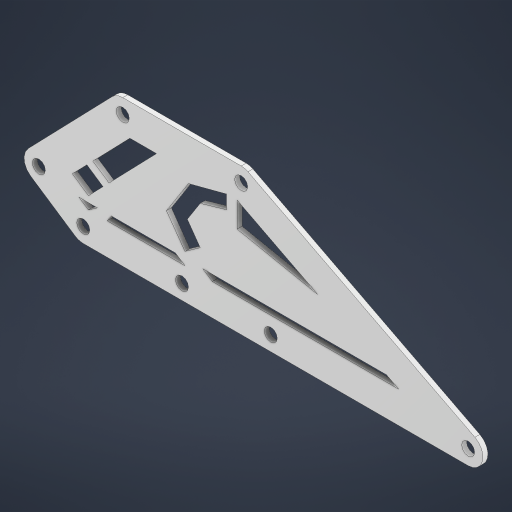
# Autodesk Inventor part: battery_mount_plate
Saved by Autodesk Inventor 2024 (Build 280153000, 153)
## iProperties
Created: 2023-11-22
Part Number: battery_mount_plate
Material: Acetal Resin, White
Document SubType Name: Modeling
Designer: avere
Density: 1.425 g/cm^3
Appearance: Smooth - White
Author: avere
Autodesk Inventor part; units mm, degrees
ref_plane "YZ Plane" through (0, 0, 0) normal (1, 0, 0) x (0, 1, 0)
ref_plane "XZ Plane" through (0, 0, 0) normal (0, 1, 0) x (-1, 0, 0)
ref_plane "XY Plane" through (0, 0, 0) normal (0, 0, 1) x (1, 0, 0)
sketch "Sketch1" plane through (0, 0, 0) normal (0, 0, 1) x (1, 0, 0)
  circle A0 centre (-66.446, -8.2221) radius 2.0955
  arc A1 (-69.8715, -4.9134) -> (-69.0877, -12.1847) centre (-66.446, -8.2221) ccw
  circle A2 centre (-39.4585, 19.7179) radius 2.0955
  circle A3 centre (-1.3585, 19.7179) radius 2.0955
  arc A4 (-39.4585, 24.4804) -> (-42.884, 23.0266) centre (-39.4585, 19.7179) ccw
  arc A5 (0.8155, 23.9553) -> (-1.3585, 24.4804) centre (-1.3585, 19.7179) ccw
  line L0 (-39.4585, 24.4804) -> (-1.3585, 24.4804)
  line L1 (-69.8715, -4.9134) -> (-42.884, 23.0266)
  circle A6 centre (-52.1585, -17.7471) radius 2.0955
  arc A7 (-54.8002, -21.7097) -> (-52.1585, -22.5096) centre (-52.1585, -17.7471) ccw
  circle A8 centre (-20.4085, -17.7471) radius 2.0955
  circle A9 centre (8.1665, -17.7471) radius 2.0955
  circle A10 centre (71.6665, -17.7471) radius 2.0955
  arc A11 (71.6665, -22.5096) -> (73.8405, -13.5097) centre (71.6665, -17.7471) ccw
  line L2 (0.8155, 23.9553) -> (73.8405, -13.5097)
  line L3 (-52.1585, -22.5096) -> (71.6665, -22.5096)
  line L4 (-54.8002, -21.7097) -> (-69.0877, -12.1847)
  line L5 (-28.575, 14.3204) -> (-37.1677, 14.3204)
  line L6 (-53.5722, -10.3176) -> (-50.5242, -12.3496)
  line L7 (-19.456, -12.3496) -> (-22.504, -10.3176)
  line L8 (-10.6535, -12.3496) -> (-13.7015, -10.3176)
  line L9 (-13.7015, -10.3176) -> (45.361, -10.3176)
  line L10 (-13.7015, -10.3176) -> (45.361, -10.3176) construction
  line L11 (-44.45, -12.3496) -> (-19.456, -12.3496)
  line L12 (-10.6535, -12.3496) -> (49.3216, -12.3496)
  line L13 (-50.5242, -12.3496) -> (-47.6187, -10.3176)
  line L14 (-44.45, -12.3496) -> (-43.0953, -10.3176)
  line L15 (-53.5722, -10.3176) -> (-47.6187, -10.3176)
  line L16 (-43.0953, -10.3176) -> (-22.504, -10.3176)
  line L17 (-53.5722, -10.3176) -> (-47.6187, -10.3176) construction
  line L18 (-43.0953, -10.3176) -> (-22.504, -10.3176) construction
  line L19 (-55.6904, -4.856) -> (-50.4835, -8.3613)
  line L20 (-51, 0) -> (-45.7931, -3.5053)
  line L21 (-49.0715, 1.9965) -> (-43.8646, -1.5088)
  line L22 (-50.4835, -8.3613) -> (-45.7931, -3.5053)
  line L23 (-43.8646, -1.5088) -> (-28.575, 14.3204)
  line L24 (-37.1677, 14.3204) -> (-49.0715, 1.9965)
  line L25 (-51, 0) -> (-55.6904, -4.856)
  line L26 (-2.6623, 14.3204) -> (-2.6623, 6.2412)
  line L27 (-2.6623, 6.2412) -> (23.3297, 0.9854)
  line L28 (23.3297, 0.9854) -> (-2.6623, 14.3204)
  line L29 (49.3216, -12.3496) -> (45.361, -10.3176)
  line L30 (-6.0786, 14.3204) -> (-18.313, 11.1125)
  line L31 (-18.313, 11.1125) -> (-25.4, 0)
  line L32 (-25.4, 0) -> (-19.456, -8.3613)
  line L33 (-19.456, -8.3613) -> (-14.5251, -4.856)
  line L34 (-14.5251, -4.856) -> (-18.6777, 0.9854)
  line L35 (-18.6777, 0.9854) -> (-14.5251, 7.4968)
  line L36 (-14.5251, 7.4968) -> (-6.0786, 9.9421)
  line L37 (-6.0786, 9.9421) -> (-6.0786, 14.3204)
  point P0 (0, 0)
  dimension "d0" = 9.525
  dimension "d1" = 9.525
  dimension "d2" = 9.525
  dimension "d3" = 9.525
  dimension "d4" = 4.191
  dimension "d5" = 4.191
  dimension "d6" = 9.525
  dimension "d9" = 10.16
  constraints: 76 end point, 12 centre point, 10 point on circle, 9 parallel, 8 tangent, 5 coincident, 3 horizontal, 2 perpendicular, 2 vertical, 5 other
  measures "d0" diameter of A1
  measures "d1" diameter of A4
  measures "d2" diameter of A5
  measures "d3" diameter of A7
  measures "d4" diameter of A8
  measures "d5" diameter of A9
  measures "d6" diameter of A11
  measures "d9" distance between parallel lines of L0 L5
extrude "Extrusion1" add sketch "Sketch1" along normal blind 1.5875
body "Solid1"
